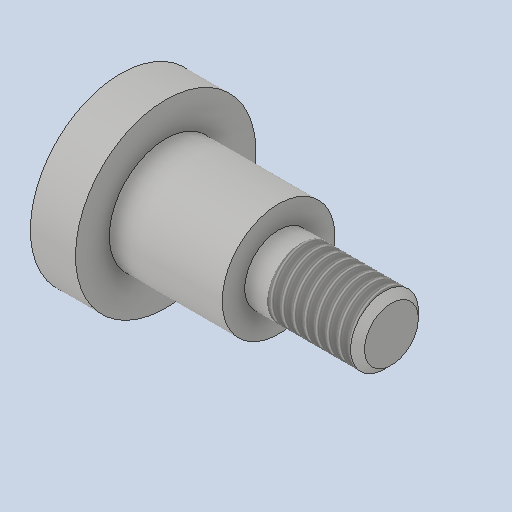
# Autodesk Inventor part: DBB3-5-5
Saved by Autodesk Inventor 2022 (Build 260153000, 153)
## iProperties
Created: 2022-10-13
Part Number: DBB3-5-5
Material: Generic
Catalog Web Link: www.cadenas.de
Description: DBB, DBM, DBS, DBSY-Stepped Screws - Low Head Selectable
Vendor: MISUMI
Document SubType Name: Modeling
Designer: psAdmin
Manufacturer: MISUMI
Mass: 0.226103 g
Surface Area: 2.88988 cm^2
Volume: 0.226103 cm^3
Density: 1 g/cm^3
Appearance: PSOLRGB-175-175-175
Category: PARTsolutions
Company: MISUMI
PSOL_IDENT_0: {$CADENAS_DATA/23d-libs/misumi/metric/27_screws_nuts/dbb.prj},182 {VTYP=3D},{NB=DBB3-5-5},{LINA=DBB3
PSOL_IDENT_1: -5-5},{NN=DBB, DBM, DBS, DBSY},{DATE=21.04.2022 12:25:58},{GEOMDATE=17.01.2022 08:24:34},{VERSION=},
PSOL_IDENT_2: {LINEID=10},{WBVAR=MAT,ST,L,F},{WBNUMERIC=L,F}  {NB=DBB3-5-5},{LINA=DBB3-5-5},{KT=DUMMY},{PN=DBB3-5-
PSOL_IDENT_3: 5},{TYPE=DB},{MAT=B},{ST=BO},{STALG= 'BO','Black Oxide','ENP','Electroless Nickel Plating' },{M=3},{
PSOL_IDENT_4: L=5},{LALG=3,4,5,6,7,8},{F=5},{FALG=3,4,5,6},{E=2.0},{DHH7=5},{A=8},{B=2.0},{LL=1.0},{HH1=2.0}
NB: DBB3-5-5
NN: DBB, DBM, DBS, DBSY
NT: Stepped Screws - Low Head Selectable
NBSYN: $PN.
LINA: DBB3-5-5
CATALOG: Misumi
PN: DBB3-5-5
TYPE: DB
MAT: 1045 Carbon Steel
ST: Black Oxide
M: 3
L: 5
F: 5
E: 2
DHH7: 5
A: 8
B: 2
LL: 1
HH1: 2
SUPPLIER: MISUMI
ARTICLENO: DBB3-5-5
BOMINFO: DBB3-5-5
CREATOR: CADENAS GmbH
Title: DBB3-5-5
Author: Cadenas PARTsolutions
Comments: Stepped Screws - Low Head Selectable
Autodesk Inventor part; units mm, degrees
ref_plane "YZ Plane" through (0, 0, 0) normal (1, 0, 0) x (0, 1, 0)
ref_plane "XZ Plane" through (0, 0, 0) normal (0, 1, 0) x (-1, 0, 0)
ref_plane "XY Plane" through (0, 0, 0) normal (0, 0, 1) x (1, 0, 0)
sketch "Sketch_1" plane through (0, 0, 0) normal (0, 0, 1) x (1, 0, 0)
  line L0 (5, 0) -> (-7, 0)
  line L1 (-7, 0) -> (-7, 4)
  line L2 (-7, 4) -> (-5, 4)
  line L3 (-5, 4) -> (-5, 2.5)
  line L4 (-5, 2.5) -> (0, 2.5)
  line L5 (0, 2.5) -> (0, 1.5)
  line L6 (0, 1.5) -> (4.6935, 1.5)
  line L7 (4.6935, 1.5) -> (5, 1.1935)
  line L8 (5, 1.1935) -> (5, 0)
  line L9 (5, 0) -> (-7, 0)
  constraints: 20 end point
revolve "Revolution1" add sketch "Sketch_1" angle 360 about axis through (5, 0, 0) along (1, 0, 0)
thread "Thread1" size "M3x0.5" class "6g" standard "ISO Metric profile" length 3.6935
sketch "Sketch_2" plane through (-7, 0, 0) normal (-1, 0, 0) x (0, 1, 0)
  line L0 (-1.1547, 0) -> (-0.5774, -1)
  line L1 (-0.5774, -1) -> (0.5774, -1)
  line L2 (0.5774, -1) -> (1.1547, 0)
  line L3 (1.1547, 0) -> (0.5774, 1)
  line L4 (0.5774, 1) -> (-0.5774, 1)
  line L5 (-0.5774, 1) -> (-1.1547, 0)
  constraints: 12 end point
extrude "Extrusion1" cut sketch "Sketch_2" against normal blind 2
sketch "Sketch_3" plane through (0, 0, 0) normal (0, 0, 1) x (1, 0, 0)
  line L0 (-4.4226, 0) -> (-5, 0)
  line L1 (-5, 0) -> (-5, 1)
  line L2 (-5, 1) -> (-4.4226, 0)
  line L3 (-4.4226, 0) -> (-5, 0)
  constraints: 8 end point
revolve "Revolution2" cut sketch "Sketch_3" angle 360 about axis through (-4.4226, 0, 0) along (1, 0, 0)
body "Solid1"
